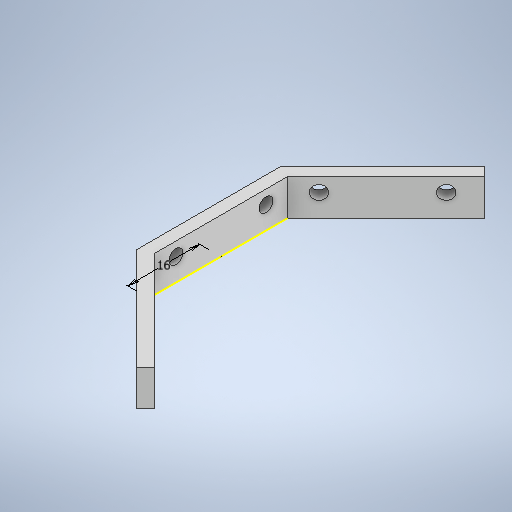
# Autodesk Inventor part: distanceSensorMount
Saved by Autodesk Inventor 2025.1 (Build 291241020, 241B)
## iProperties
Created: 2025-04-15
Part Number: distanceSensorMount
Material: Generic
Document SubType Name: Modeling
Designer: 7008661
Density: 1 g/cm^3
Appearance: Default
Author: 7008661
Autodesk Inventor part; units mm, degrees
ref_plane "YZ Plane" through (0, 0, 0) normal (1, 0, 0) x (0, 1, 0)
ref_plane "XZ Plane" through (0, 0, 0) normal (0, 1, 0) x (-1, 0, 0)
ref_plane "XY Plane" through (0, 0, 0) normal (0, 0, 1) x (1, 0, 0)
sketch "Sketch1" plane through (0, 0, 0) normal (0, 1, 0) x (-1, 0, 0)
  line L0 (-6.364, 4.3033) -> (-6.364, 17.3033)
  line L1 (-6.364, 4.3033) -> (-6.364, -8.6967)
  line L2 (-6.364, 17.3033) -> (-6.364, 20.3033)
  line L3 (-3.6569, 19.6569) -> (-26.2843, 42.2843)
  line L4 (-26.2843, 42.2843) -> (-27.6985, 40.8701)
  line L5 (-3.6569, -9.3431) -> (-3.6569, -12.3431)
  line L6 (-3.6569, -12.3431) -> (-26.2843, -34.9706)
  line L7 (-26.2843, -34.9706) -> (-28.2843, -32.9706)
  line L8 (-28.2843, -32.9706) -> (-6.364, -11.0503)
  line L9 (-6.364, -11.0503) -> (-6.364, -8.6967)
  line L10 (-3.6569, 19.6569) -> (-3.6569, -12.3431)
  line L11 (-3.6569, -12.3431) -> (-26.2843, -34.9706)
  line L12 (-28.2843, -32.9706) -> (-26.2843, -34.9706)
  line L13 (-28.2843, -32.9706) -> (-6.364, -11.0503)
  line L14 (-6.364, -11.0503) -> (-6.364, 19.5355)
  line L15 (-27.6985, 40.8701) -> (-26.2843, 42.2843)
  line L16 (-26.2843, 42.2843) -> (-3.6569, 19.6569)
  line L17 (-3.6569, 19.6569) -> (-0.6568, 19.6569) construction
  line L18 (-6.364, 18.3639) -> (-28.2843, 40.2842) construction
  line L19 (-28.2843, 40.2842) -> (-26.2843, 42.2843) construction
  line L20 (-26.2843, 42.2843) -> (-28.2843, 40.2842)
  line L21 (-6.364, 18.3639) -> (-28.2843, 40.2842)
  point P0 (0, 0)
  dimension "d64" = 32
  dimension "d65" = 32
  dimension "d66" = 2
  dimension "d67" = 32
  dimension "d70" = 31
  constraints: 44 end point, 7 collinear, 6 perpendicular, 3 point on line, 3 vertical, 1 horizontal, 1 parallel
  measures "d64" distance of L5.end L6.end
  measures "d65" distance of L3.start L3.end
  measures "d66" horizontal distance of L6.end L7.end
  measures "d67" distance of L3.start L5.end
  measures "d70" distance of L7.end L8.end
extrude "Extrusion2" add sketch "Sketch1" along normal blind 8
sketch "Sketch9" plane through (3.6569, 0, -12.3431) normal (-1, 0, 0) x (0, 0, 1)
  line L0 (0, 0) -> (0, 8) projected
  line L1 (0, 8) -> (32, 8) projected
  line L2 (0, 8) -> (32, 8)
  line L3 (0, 8) -> (16, 8)
  line L4 (16, 8) -> (32, 8)
  line L5 (16, 8) -> (16, 0)
  line L6 (16, 0) -> (3, 0)
  line L7 (30.707, 0) -> (1.2929, 0) projected
  line L8 (3, 0) -> (6, 0)
  line L9 (6, 0) -> (6, 5)
  line L10 (6, 5) -> (16, 5)
  line L11 (16, 5) -> (26, 5)
  line L12 (26, 5) -> (26, 0)
  circle A0 centre (6, 5) radius 1.525
  circle A1 centre (26, 5) radius 1.525
  point P0 (12.3431, 0)
  dimension "d72" = 16
  dimension "d73" = 13
  dimension "d74" = 3
  dimension "d75" = 5
  dimension "d76" = 10
  dimension "d77" = 3.05
  dimension "d78" = 3.05
  constraints: 20 end point, 4 point on line, 3 perpendicular, 2 centre point, 2 coincident, 2 collinear, 1 horizontal, 1 midpoint, 1 vertical
  measures "d72" distance of L0.end L3.end
  measures "d73" distance of L5.end L6.end
  measures "d74" distance of L6.end L8.end
  measures "d75" distance of L8.end L9.end
  measures "d76" distance of L10.end L11.end
  measures "d77" diameter of A0
  measures "d78" diameter of A1
extrude "Extrusion7" cut sketch "Sketch9" against normal blind 8 contours A0 L9 L10 | L10 L9 A0 | A1 L12 L11 | L11 L12 A1
sketch "Sketch10" plane through (3.6569, 0, -12.3431) normal (-0.7071068, 0, -0.7071068) x (-0.7071068, 0, 0.7071068)
  line L0 (-32, 0) -> (0, 0) projected
  line L1 (-16, 0) -> (-32, 0)
  line L2 (-32, 0) -> (-16, 0)
  line L3 (0, 0) -> (-16, 0)
  line L4 (-16, 0) -> (-29, 0)
  line L5 (-29, 0) -> (-26, 0)
  line L6 (-26, 0) -> (-26, 5)
  line L7 (-26, 5) -> (-16, 5)
  line L8 (-16, 5) -> (-6, 5)
  line L9 (-6, 5) -> (-6, 0)
  circle A0 centre (-26, 5) radius 1.525
  circle A1 centre (-6, 5) radius 1.525
  point P0 (11.3137, 0)
  dimension "d81" = 13
  dimension "d82" = 3
  dimension "d83" = 5
  dimension "d84" = 10
  dimension "d85" = 3.05
  dimension "d86" = 3.05
  constraints: 18 end point, 4 point on line, 3 collinear, 3 perpendicular, 2 centre point, 2 coincident, 1 midpoint
  measures "d81" distance of L1.start L4.end
  measures "d82" distance of L4.end L5.end
  measures "d83" distance of L5.end L6.end
  measures "d84" distance of L7.end L8.end
  measures "d85" diameter of A0
  measures "d86" diameter of A1
extrude "Extrusion8" cut sketch "Sketch10" against normal blind 8 contours A0 L7 L6 | L6 L7 A0 | A1 L8 L9 | L9 L8 A1
sketch "Sketch11" plane through (26.2843, 0, 42.2843) normal (-0.7071068, 0, 0.7071068) x (0.7071068, 0, 0.7071068)
  line L0 (-32, 0) -> (-32, 8) projected
  line L1 (-32, 0) -> (0, 0) projected
  line L2 (-32, 0) -> (0, 0)
  line L3 (0, 0) -> (-16, 0)
  line L4 (-16, 0) -> (-32, 0)
  line L5 (-16, 0) -> (-29, 0)
  line L6 (0, 0) -> (-31.0001, 0) projected
  line L7 (-29, 0) -> (-26, 0)
  line L8 (-26, 0) -> (-26, 5)
  line L9 (-26, 5) -> (-16, 5)
  line L10 (-16, 5) -> (-6, 5)
  line L11 (-6, 5) -> (-6, 0)
  circle A0 centre (-26, 5) radius 1.525
  circle A1 centre (-6, 5) radius 1.525
  point P0 (-48.4853, 0)
  dimension "d89" = 16
  dimension "d90" = 13
  dimension "d91" = 3
  dimension "d92" = 5
  dimension "d93" = 10
  dimension "d94" = 3.05
  dimension "d95" = 3.05
  constraints: 18 end point, 4 point on line, 3 perpendicular, 2 centre point, 2 coincident, 2 collinear, 1 midpoint
  measures "d89" distance of L1.end L3.end
  measures "d90" distance of L3.end L5.end
  measures "d91" distance of L5.end L7.end
  measures "d92" distance of L7.end L8.end
  measures "d93" distance of L9.end L10.end
  measures "d94" diameter of A0
  measures "d95" diameter of A1
extrude "Extrusion9" cut sketch "Sketch11" against normal blind 8 contours A0 L9 L8 | L8 L9 A0 | A1 L10 L11 | L11 L10 A1
sketch "Sketch12" plane through (0, 0, 0) normal (0, -1, 0) x (1, 0, 0)
  line L0 (3.6569, -12.3431) -> (3.6569, 19.6569) projected
  line L1 (3.6569, -12.3431) -> (3.6569, 19.6569)
  line L2 (3.6569, 19.6569) -> (3.6569, 3.6569)
  line L3 (3.6569, 3.6569) -> (6.364, 3.6568)
  line L4 (6.364, 18.3639) -> (6.364, -11.0503) projected
  point P0 (0, 0)
  dimension "d98" = 16
  constraints: 6 end point, 2 midpoint, 1 collinear
  measures "d98" distance of L0.end L2.end
body "Solid2"
